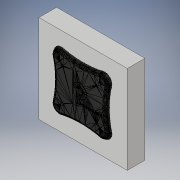
# Autodesk Inventor part: LpmsB2
Saved by Autodesk Inventor 2019.4 (Build 234330000, 330)
## iProperties
Created: 2021-05-02
Part Number: LpmsB2
Material: Generic
Document SubType Name: Modeling
Designer: mx19
Density: 1 g/cm^3
Appearance: Default
Author: mx19
Autodesk Inventor part; units mm, degrees
ref_plane "YZ Plane" through (0, 0, 0) normal (1, 0, 0) x (0, 1, 0)
ref_plane "XZ Plane" through (0, 0, 0) normal (0, 1, 0) x (-1, 0, 0)
ref_plane "XY Plane" through (0, 0, 0) normal (0, 0, 1) x (1, 0, 0)
sketch "Sketch1" plane through (0, 0, 0) normal (0, 0, 1) x (1, 0, 0)
  line L0 (-2584.9626, 861.4042) -> (-1084.9626, 861.4042)
  line L1 (-1084.9626, 861.4042) -> (-1084.9626, -638.5958)
  line L2 (-1084.9626, -638.5958) -> (-2584.9626, -638.5958)
  line L3 (-2584.9626, -638.5958) -> (-2584.9626, 861.4042)
  point P0 (0, 0)
  dimension "d0" = 1500
  dimension "d1" = 1500
  constraints: 8 end point, 2 parallel, 1 horizontal, 1 perpendicular
  measures "d0" distance of L1.end L2.end
  measures "d1" distance of L0.end L1.end
extrude "Extrusion1" add sketch "Sketch1" along normal blind 100 and the other way blind 200
body "Solid1"
